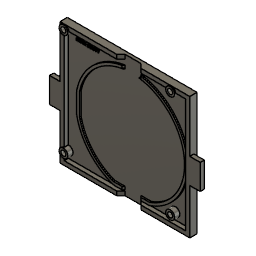
pin_grid_wafer_jig_sla (Autodesk Fusion 360 design; units mm, degrees)
part number: 2026-08-12-03-32-45-867
Autodesk Fusion 360 part; units mm, degrees
ref_plane "WorkPlane1" through (0, 0, 3) normal (0, 0, 1) x (1, 0, 0)
ref_plane "WorkPlane2" through (0, 0, 4.7) normal (0, 0, 1) x (1, 0, 0)
ref_plane "WorkPlane3" through (0, 0, 7.2) normal (0, 0, 1) x (1, 0, 0)
ref_plane "WorkPlane4" through (0, 0, 8) normal (0, 0, 1) x (1, 0, 0)
sketch "Wafer Platform Sketch" plane through (0, 0, 0) normal (0, 0, 1) x (1, 0, 0)
  line L0 (-55.05, -61.5817) -> (68.477, -61.5817)
  line L1 (68.477, -61.5817) -> (68.477, 55.05)
  line L2 (68.477, 55.05) -> (-55.05, 55.05)
  line L3 (-55.05, 55.05) -> (-55.05, -61.5817)
extrude "Wafer Platform" add sketch "Wafer Platform Sketch" along normal blind 3
sketch "4 x 4 mm Perimeter Reinforcement Bar Sketch" plane through (0, 0, 3) normal (0, 0, 1) x (1, 0, 0)
  line L0 (-55.05, -61.5817) -> (68.477, -61.5817)
  line L1 (68.477, -61.5817) -> (68.477, 55.05)
  line L2 (68.477, 55.05) -> (-55.05, 55.05)
  line L3 (-55.05, 55.05) -> (-55.05, -61.5817)
  line L4 (-51.05, -57.5817) -> (64.477, -57.5817)
  line L5 (64.477, -57.5817) -> (64.477, 51.05)
  line L6 (64.477, 51.05) -> (-51.05, 51.05)
  line L7 (-51.05, 51.05) -> (-51.05, -57.5817)
extrude "4 x 4 mm Perimeter Reinforcement Bar" add sketch "4 x 4 mm Perimeter Reinforcement Bar Sketch" along normal blind 4
sketch "Left Pickup Tab Sketch" plane through (0, 0, 3) normal (0, 0, 1) x (1, 0, 0)
  line L0 (-65.05, -18.296) -> (-55.05, -18.296)
  line L1 (-55.05, -18.296) -> (-55.05, 5.704)
  line L2 (-55.05, 5.704) -> (-65.05, 5.704)
  line L3 (-65.05, 5.704) -> (-65.05, -18.296)
extrude "Left Pickup Tab" add sketch "Left Pickup Tab Sketch" along normal blind 4
sketch "Right Pickup Tab Sketch" plane through (0, 0, 3) normal (0, 0, 1) x (1, 0, 0)
  line L0 (68.477, -18.296) -> (78.477, -18.296)
  line L1 (78.477, -18.296) -> (78.477, 5.704)
  line L2 (78.477, 5.704) -> (68.477, 5.704)
  line L3 (68.477, 5.704) -> (68.477, -18.296)
extrude "Right Pickup Tab" add sketch "Right Pickup Tab Sketch" along normal blind 4
sketch "15 mm Outer Bar Tweezer Notch with 45 Degree Sides Lower Sketch" plane through (0, 0, 3) normal (0, 0, 1) x (1, 0, 0)
  line L0 (2.977, -61.6817) -> (17.977, -61.6817)
  line L1 (17.977, -61.6817) -> (17.977, -57.4817)
  line L2 (17.977, -57.4817) -> (2.977, -57.4817)
  line L3 (2.977, -57.4817) -> (2.977, -61.6817)
sketch "15 mm Outer Bar Tweezer Notch with 45 Degree Sides Upper Sketch" plane through (0, 0, 7.2) normal (0, 0, 1) x (1, 0, 0)
  line L0 (-1.223, -65.8817) -> (22.177, -65.8817)
  line L1 (22.177, -65.8817) -> (22.177, -53.2817)
  line L2 (22.177, -53.2817) -> (-1.223, -53.2817)
  line L3 (-1.223, -53.2817) -> (-1.223, -65.8817)
loft "15 mm Outer Bar Tweezer Notch with 45 Degree Sides" cut profiles "15 mm Outer Bar Tweezer Notch with 45 Degree Sides Lower Sketch", "15 mm Outer Bar Tweezer Notch with 45 Degree Sides Upper Sketch" section 1 section 2
sketch "1.5 mm Raised Wafer Nest Sketch" plane through (0, 0, 3) normal (0, 0, 1) x (1, 0, 0)
  line L0 (63.477, -6.296) -> (63.4447, -4.4463)
  line L1 (63.4447, -4.4463) -> (63.3479, -2.5989)
  line L2 (63.3479, -2.5989) -> (63.1867, -0.756)
  line L3 (63.1867, -0.756) -> (62.9612, 1.0802)
  line L4 (62.9612, 1.0802) -> (62.6718, 2.9074)
  line L5 (62.6718, 2.9074) -> (62.3188, 4.7233)
  line L6 (62.3188, 4.7233) -> (61.9027, 6.5259)
  line L7 (61.9027, 6.5259) -> (61.4239, 8.3128)
  line L8 (61.4239, 8.3128) -> (60.883, 10.0819)
  line L9 (60.883, 10.0819) -> (60.2807, 11.8311)
  line L10 (60.2807, 11.8311) -> (59.6177, 13.5581)
  line L11 (59.6177, 13.5581) -> (58.8949, 15.261)
  line L12 (58.8949, 15.261) -> (58.1131, 16.9377)
  line L13 (58.1131, 16.9377) -> (57.2732, 18.586)
  line L14 (57.2732, 18.586) -> (56.3763, 20.204)
  line L15 (56.3763, 20.204) -> (55.4235, 21.7897)
  line L16 (55.4235, 21.7897) -> (54.416, 23.3412)
  line L17 (54.416, 23.3412) -> (53.3549, 24.8566)
  line L18 (53.3549, 24.8566) -> (52.2416, 26.3341)
  line L19 (52.2416, 26.3341) -> (51.0774, 27.7717)
  line L20 (51.0774, 27.7717) -> (49.8637, 29.1679)
  line L21 (49.8637, 29.1679) -> (48.602, 30.5209)
  line L22 (48.602, 30.5209) -> (47.2939, 31.829)
  line L23 (47.2939, 31.829) -> (45.9409, 33.0907)
  line L24 (45.9409, 33.0907) -> (44.5447, 34.3044)
  line L25 (44.5447, 34.3044) -> (43.1071, 35.4686)
  line L26 (43.1071, 35.4686) -> (41.6296, 36.5819)
  line L27 (41.6296, 36.5819) -> (40.1142, 37.643)
  line L28 (40.1142, 37.643) -> (38.5627, 38.6505)
  line L29 (38.5627, 38.6505) -> (36.977, 39.6033)
  line L30 (36.977, 39.6033) -> (35.359, 40.5002)
  line L31 (35.359, 40.5002) -> (33.7107, 41.3401)
  line L32 (33.7107, 41.3401) -> (32.034, 42.1219)
  line L33 (32.034, 42.1219) -> (30.3311, 42.8447)
  line L34 (30.3311, 42.8447) -> (28.6041, 43.5077)
  line L35 (28.6041, 43.5077) -> (26.8549, 44.11)
  line L36 (26.8549, 44.11) -> (25.0858, 44.6509)
  line L37 (25.0858, 44.6509) -> (23.2989, 45.1297)
  line L38 (23.2989, 45.1297) -> (21.4963, 45.5458)
  line L39 (21.4963, 45.5458) -> (19.6804, 45.8988)
  line L40 (19.6804, 45.8988) -> (17.8532, 46.1882)
  line L41 (17.8532, 46.1882) -> (16.017, 46.4137)
  line L42 (16.017, 46.4137) -> (14.1741, 46.5749)
  line L43 (14.1741, 46.5749) -> (12.3267, 46.6717)
  line L44 (12.3267, 46.6717) -> (10.477, 46.704)
  line L45 (10.477, 46.704) -> (8.6273, 46.6717)
  line L46 (8.6273, 46.6717) -> (6.7799, 46.5749)
  line L47 (6.7799, 46.5749) -> (4.937, 46.4137)
  line L48 (4.937, 46.4137) -> (3.1008, 46.1882)
  line L49 (3.1008, 46.1882) -> (1.2736, 45.8988)
  line L50 (1.2736, 45.8988) -> (-0.5423, 45.5458)
  line L51 (-0.5423, 45.5458) -> (-2.3449, 45.1297)
  line L52 (-2.3449, 45.1297) -> (-4.1318, 44.6509)
  line L53 (-4.1318, 44.6509) -> (-5.9009, 44.11)
  line L54 (-5.9009, 44.11) -> (-7.6501, 43.5077)
  line L55 (-7.6501, 43.5077) -> (-9.3771, 42.8447)
  line L56 (-9.3771, 42.8447) -> (-11.08, 42.1219)
  line L57 (-11.08, 42.1219) -> (-12.7567, 41.3401)
  line L58 (-12.7567, 41.3401) -> (-14.405, 40.5002)
  line L59 (-14.405, 40.5002) -> (-16.023, 39.6033)
  line L60 (-16.023, 39.6033) -> (-17.6087, 38.6505)
  line L61 (-17.6087, 38.6505) -> (-19.1602, 37.643)
  line L62 (-19.1602, 37.643) -> (-20.6756, 36.5819)
  line L63 (-20.6756, 36.5819) -> (-22.1531, 35.4686)
  line L64 (-22.1531, 35.4686) -> (-23.5907, 34.3044)
  line L65 (-23.5907, 34.3044) -> (-24.9869, 33.0907)
  line L66 (-24.9869, 33.0907) -> (-26.3399, 31.829)
  line L67 (-26.3399, 31.829) -> (-27.648, 30.5209)
  line L68 (-27.648, 30.5209) -> (-28.9097, 29.1679)
  line L69 (-28.9097, 29.1679) -> (-30.1234, 27.7717)
  line L70 (-30.1234, 27.7717) -> (-31.2876, 26.3341)
  line L71 (-31.2876, 26.3341) -> (-32.4009, 24.8566)
  line L72 (-32.4009, 24.8566) -> (-33.462, 23.3412)
  line L73 (-33.462, 23.3412) -> (-34.4695, 21.7897)
  line L74 (-34.4695, 21.7897) -> (-35.4223, 20.204)
  line L75 (-35.4223, 20.204) -> (-36.3192, 18.586)
  line L76 (-36.3192, 18.586) -> (-37.1591, 16.9377)
  line L77 (-37.1591, 16.9377) -> (-37.9409, 15.261)
  line L78 (-37.9409, 15.261) -> (-38.6637, 13.5581)
  line L79 (-38.6637, 13.5581) -> (-39.3267, 11.8311)
  line L80 (-39.3267, 11.8311) -> (-39.929, 10.0819)
  line L81 (-39.929, 10.0819) -> (-40.4699, 8.3128)
  line L82 (-40.4699, 8.3128) -> (-40.9487, 6.5259)
  line L83 (-40.9487, 6.5259) -> (-41.3648, 4.7233)
  line L84 (-41.3648, 4.7233) -> (-41.7063, 2.9664)
  line L85 (-41.7063, 2.9664) -> (-41.7063, -15.5584)
  line L86 (-41.7063, -15.5584) -> (-41.3648, -17.3153)
  line L87 (-41.3648, -17.3153) -> (-40.9487, -19.1179)
  line L88 (-40.9487, -19.1179) -> (-40.4699, -20.9048)
  line L89 (-40.4699, -20.9048) -> (-39.929, -22.6739)
  line L90 (-39.929, -22.6739) -> (-39.3267, -24.4231)
  line L91 (-39.3267, -24.4231) -> (-38.6637, -26.1501)
  line L92 (-38.6637, -26.1501) -> (-37.9409, -27.853)
  line L93 (-37.9409, -27.853) -> (-37.1591, -29.5297)
  line L94 (-37.1591, -29.5297) -> (-36.3192, -31.178)
  line L95 (-36.3192, -31.178) -> (-35.4223, -32.796)
  line L96 (-35.4223, -32.796) -> (-34.4695, -34.3817)
  line L97 (-34.4695, -34.3817) -> (-33.462, -35.9332)
  line L98 (-33.462, -35.9332) -> (-32.4009, -37.4486)
  line L99 (-32.4009, -37.4486) -> (-31.2876, -38.9261)
  line L100 (-31.2876, -38.9261) -> (-30.1234, -40.3637)
  line L101 (-30.1234, -40.3637) -> (-28.9097, -41.7599)
  line L102 (-28.9097, -41.7599) -> (-27.648, -43.1129)
  line L103 (-27.648, -43.1129) -> (-26.3399, -44.421)
  line L104 (-26.3399, -44.421) -> (-24.9869, -45.6827)
  line L105 (-24.9869, -45.6827) -> (-23.5907, -46.8964)
  line L106 (-23.5907, -46.8964) -> (-22.1531, -48.0606)
  line L107 (-22.1531, -48.0606) -> (-20.6756, -49.1739)
  line L108 (-20.6756, -49.1739) -> (-19.1602, -50.235)
  line L109 (-19.1602, -50.235) -> (-17.6087, -51.2425)
  line L110 (-17.6087, -51.2425) -> (-16.023, -52.1953)
  line L111 (-16.023, -52.1953) -> (-14.405, -53.0922)
  line L112 (-14.405, -53.0922) -> (-12.7567, -53.9321)
  line L113 (-12.7567, -53.9321) -> (-11.08, -54.7139)
  line L114 (-11.08, -54.7139) -> (-9.3771, -55.4367)
  line L115 (-9.3771, -55.4367) -> (-7.6501, -56.0997)
  line L116 (-7.6501, -56.0997) -> (-6.2503, -56.5817)
  line L117 (-6.2503, -56.5817) -> (27.2043, -56.5817)
  line L118 (27.2043, -56.5817) -> (28.6041, -56.0997)
  line L119 (28.6041, -56.0997) -> (30.3311, -55.4367)
  line L120 (30.3311, -55.4367) -> (32.034, -54.7139)
  line L121 (32.034, -54.7139) -> (33.7107, -53.9321)
  line L122 (33.7107, -53.9321) -> (35.359, -53.0922)
  line L123 (35.359, -53.0922) -> (36.977, -52.1953)
  line L124 (36.977, -52.1953) -> (38.5627, -51.2425)
  line L125 (38.5627, -51.2425) -> (40.1142, -50.235)
  line L126 (40.1142, -50.235) -> (41.6296, -49.1739)
  line L127 (41.6296, -49.1739) -> (43.1071, -48.0606)
  line L128 (43.1071, -48.0606) -> (44.5447, -46.8964)
  line L129 (44.5447, -46.8964) -> (45.9409, -45.6827)
  line L130 (45.9409, -45.6827) -> (47.2939, -44.421)
  line L131 (47.2939, -44.421) -> (48.602, -43.1129)
  line L132 (48.602, -43.1129) -> (49.8637, -41.7599)
  line L133 (49.8637, -41.7599) -> (51.0774, -40.3637)
  line L134 (51.0774, -40.3637) -> (52.2416, -38.9261)
  line L135 (52.2416, -38.9261) -> (53.3549, -37.4486)
  line L136 (53.3549, -37.4486) -> (54.416, -35.9332)
  line L137 (54.416, -35.9332) -> (55.4235, -34.3817)
  line L138 (55.4235, -34.3817) -> (56.3763, -32.796)
  line L139 (56.3763, -32.796) -> (57.2732, -31.178)
  line L140 (57.2732, -31.178) -> (58.1131, -29.5297)
  line L141 (58.1131, -29.5297) -> (58.8949, -27.853)
  line L142 (58.8949, -27.853) -> (59.6177, -26.1501)
  line L143 (59.6177, -26.1501) -> (60.2807, -24.4231)
  line L144 (60.2807, -24.4231) -> (60.883, -22.6739)
  line L145 (60.883, -22.6739) -> (61.4239, -20.9048)
  line L146 (61.4239, -20.9048) -> (61.9027, -19.1179)
  line L147 (61.9027, -19.1179) -> (62.3188, -17.3153)
  line L148 (62.3188, -17.3153) -> (62.6718, -15.4994)
  line L149 (62.6718, -15.4994) -> (62.9612, -13.6722)
  line L150 (62.9612, -13.6722) -> (63.1867, -11.836)
  line L151 (63.1867, -11.836) -> (63.3479, -9.9931)
  line L152 (63.3479, -9.9931) -> (63.4447, -8.1457)
  line L153 (63.4447, -8.1457) -> (63.477, -6.296)
extrude "1.5 mm Raised Wafer Nest" add sketch "1.5 mm Raised Wafer Nest Sketch" along normal blind 1.5
sketch "Final Wafer Pocket Clearance Sketch" plane through (0, 0, 3) normal (0, 0, 1) x (1, 0, 0)
  line L0 (60.977, -6.296) -> (60.9462, -4.5336)
  line L1 (60.9462, -4.5336) -> (60.854, -2.7733)
  line L2 (60.854, -2.7733) -> (60.7004, -1.0173)
  line L3 (60.7004, -1.0173) -> (60.4855, 0.7322)
  line L4 (60.4855, 0.7322) -> (60.2098, 2.4732)
  line L5 (60.2098, 2.4732) -> (59.8735, 4.2035)
  line L6 (59.8735, 4.2035) -> (59.4769, 5.9211)
  line L7 (59.4769, 5.9211) -> (59.0207, 7.6237)
  line L8 (59.0207, 7.6237) -> (58.5054, 9.3094)
  line L9 (58.5054, 9.3094) -> (57.9315, 10.976)
  line L10 (57.9315, 10.976) -> (57.2998, 12.6216)
  line L11 (57.2998, 12.6216) -> (56.611, 14.2442)
  line L12 (56.611, 14.2442) -> (55.8661, 15.8417)
  line L13 (55.8661, 15.8417) -> (55.0659, 17.4123)
  line L14 (55.0659, 17.4123) -> (54.2113, 18.954)
  line L15 (54.2113, 18.954) -> (53.3034, 20.4649)
  line L16 (53.3034, 20.4649) -> (52.3434, 21.9432)
  line L17 (52.3434, 21.9432) -> (51.3324, 23.3872)
  line L18 (51.3324, 23.3872) -> (50.2715, 24.7949)
  line L19 (50.2715, 24.7949) -> (49.1622, 26.1648)
  line L20 (49.1622, 26.1648) -> (48.0058, 27.4951)
  line L21 (48.0058, 27.4951) -> (46.8037, 28.7842)
  line L22 (46.8037, 28.7842) -> (45.5572, 30.0307)
  line L23 (45.5572, 30.0307) -> (44.2681, 31.2328)
  line L24 (44.2681, 31.2328) -> (42.9378, 32.3892)
  line L25 (42.9378, 32.3892) -> (41.5679, 33.4985)
  line L26 (41.5679, 33.4985) -> (40.1602, 34.5594)
  line L27 (40.1602, 34.5594) -> (38.7162, 35.5704)
  line L28 (38.7162, 35.5704) -> (37.2379, 36.5304)
  line L29 (37.2379, 36.5304) -> (35.727, 37.4383)
  line L30 (35.727, 37.4383) -> (34.1853, 38.2929)
  line L31 (34.1853, 38.2929) -> (32.6147, 39.0931)
  line L32 (32.6147, 39.0931) -> (31.0172, 39.838)
  line L33 (31.0172, 39.838) -> (29.3946, 40.5268)
  line L34 (29.3946, 40.5268) -> (27.749, 41.1585)
  line L35 (27.749, 41.1585) -> (26.0824, 41.7324)
  line L36 (26.0824, 41.7324) -> (24.3967, 42.2477)
  line L37 (24.3967, 42.2477) -> (22.6941, 42.7039)
  line L38 (22.6941, 42.7039) -> (20.9765, 43.1005)
  line L39 (20.9765, 43.1005) -> (19.2462, 43.4368)
  line L40 (19.2462, 43.4368) -> (17.5052, 43.7125)
  line L41 (17.5052, 43.7125) -> (15.7557, 43.9274)
  line L42 (15.7557, 43.9274) -> (13.9997, 44.081)
  line L43 (13.9997, 44.081) -> (12.2394, 44.1732)
  line L44 (12.2394, 44.1732) -> (10.477, 44.204)
  line L45 (10.477, 44.204) -> (8.7146, 44.1732)
  line L46 (8.7146, 44.1732) -> (6.9543, 44.081)
  line L47 (6.9543, 44.081) -> (5.1983, 43.9274)
  line L48 (5.1983, 43.9274) -> (3.4488, 43.7125)
  line L49 (3.4488, 43.7125) -> (1.7078, 43.4368)
  line L50 (1.7078, 43.4368) -> (-0.0225, 43.1005)
  line L51 (-0.0225, 43.1005) -> (-1.7401, 42.7039)
  line L52 (-1.7401, 42.7039) -> (-3.4427, 42.2477)
  line L53 (-3.4427, 42.2477) -> (-5.1284, 41.7324)
  line L54 (-5.1284, 41.7324) -> (-6.795, 41.1585)
  line L55 (-6.795, 41.1585) -> (-8.4406, 40.5268)
  line L56 (-8.4406, 40.5268) -> (-10.0632, 39.838)
  line L57 (-10.0632, 39.838) -> (-11.6607, 39.0931)
  line L58 (-11.6607, 39.0931) -> (-13.2313, 38.2929)
  line L59 (-13.2313, 38.2929) -> (-14.773, 37.4383)
  line L60 (-14.773, 37.4383) -> (-16.2839, 36.5304)
  line L61 (-16.2839, 36.5304) -> (-17.7622, 35.5704)
  line L62 (-17.7622, 35.5704) -> (-19.2062, 34.5594)
  line L63 (-19.2062, 34.5594) -> (-20.6139, 33.4985)
  line L64 (-20.6139, 33.4985) -> (-21.9838, 32.3892)
  line L65 (-21.9838, 32.3892) -> (-23.3141, 31.2328)
  line L66 (-23.3141, 31.2328) -> (-24.6032, 30.0307)
  line L67 (-24.6032, 30.0307) -> (-25.8497, 28.7842)
  line L68 (-25.8497, 28.7842) -> (-27.0518, 27.4951)
  line L69 (-27.0518, 27.4951) -> (-28.2082, 26.1648)
  line L70 (-28.2082, 26.1648) -> (-29.3175, 24.7949)
  line L71 (-29.3175, 24.7949) -> (-30.3784, 23.3872)
  line L72 (-30.3784, 23.3872) -> (-31.3894, 21.9432)
  line L73 (-31.3894, 21.9432) -> (-32.3494, 20.4649)
  line L74 (-32.3494, 20.4649) -> (-33.2573, 18.954)
  line L75 (-33.2573, 18.954) -> (-34.1119, 17.4123)
  line L76 (-34.1119, 17.4123) -> (-34.9121, 15.8417)
  line L77 (-34.9121, 15.8417) -> (-35.657, 14.2442)
  line L78 (-35.657, 14.2442) -> (-36.3458, 12.6216)
  line L79 (-36.3458, 12.6216) -> (-36.9775, 10.976)
  line L80 (-36.9775, 10.976) -> (-37.5514, 9.3094)
  line L81 (-37.5514, 9.3094) -> (-38.0667, 7.6237)
  line L82 (-38.0667, 7.6237) -> (-38.5229, 5.9211)
  line L83 (-38.5229, 5.9211) -> (-38.8813, 4.3687)
  line L84 (-38.8813, 4.3687) -> (-38.8813, -16.9607)
  line L85 (-38.8813, -16.9607) -> (-38.5229, -18.5131)
  line L86 (-38.5229, -18.5131) -> (-38.0667, -20.2157)
  line L87 (-38.0667, -20.2157) -> (-37.5514, -21.9014)
  line L88 (-37.5514, -21.9014) -> (-36.9775, -23.568)
  line L89 (-36.9775, -23.568) -> (-36.3458, -25.2136)
  line L90 (-36.3458, -25.2136) -> (-35.657, -26.8362)
  line L91 (-35.657, -26.8362) -> (-34.9121, -28.4337)
  line L92 (-34.9121, -28.4337) -> (-34.1119, -30.0043)
  line L93 (-34.1119, -30.0043) -> (-33.2573, -31.546)
  line L94 (-33.2573, -31.546) -> (-32.3494, -33.0569)
  line L95 (-32.3494, -33.0569) -> (-31.3894, -34.5352)
  line L96 (-31.3894, -34.5352) -> (-30.3784, -35.9792)
  line L97 (-30.3784, -35.9792) -> (-29.3175, -37.3869)
  line L98 (-29.3175, -37.3869) -> (-28.2082, -38.7568)
  line L99 (-28.2082, -38.7568) -> (-27.0518, -40.0871)
  line L100 (-27.0518, -40.0871) -> (-25.8497, -41.3762)
  line L101 (-25.8497, -41.3762) -> (-24.6032, -42.6227)
  line L102 (-24.6032, -42.6227) -> (-23.3141, -43.8248)
  line L103 (-23.3141, -43.8248) -> (-21.9838, -44.9812)
  line L104 (-21.9838, -44.9812) -> (-20.6139, -46.0905)
  line L105 (-20.6139, -46.0905) -> (-19.2062, -47.1514)
  line L106 (-19.2062, -47.1514) -> (-17.7622, -48.1624)
  line L107 (-17.7622, -48.1624) -> (-16.2839, -49.1224)
  line L108 (-16.2839, -49.1224) -> (-14.773, -50.0303)
  line L109 (-14.773, -50.0303) -> (-13.2313, -50.8849)
  line L110 (-13.2313, -50.8849) -> (-11.6607, -51.6851)
  line L111 (-11.6607, -51.6851) -> (-10.0632, -52.43)
  line L112 (-10.0632, -52.43) -> (-8.4406, -53.1188)
  line L113 (-8.4406, -53.1188) -> (-6.795, -53.7505)
  line L114 (-6.795, -53.7505) -> (-6.7769, -53.7567)
  line L115 (-6.7769, -53.7567) -> (27.7309, -53.7567)
  line L116 (27.7309, -53.7567) -> (27.749, -53.7505)
  line L117 (27.749, -53.7505) -> (29.3946, -53.1188)
  line L118 (29.3946, -53.1188) -> (31.0172, -52.43)
  line L119 (31.0172, -52.43) -> (32.6147, -51.6851)
  line L120 (32.6147, -51.6851) -> (34.1853, -50.8849)
  line L121 (34.1853, -50.8849) -> (35.727, -50.0303)
  line L122 (35.727, -50.0303) -> (37.2379, -49.1224)
  line L123 (37.2379, -49.1224) -> (38.7162, -48.1624)
  line L124 (38.7162, -48.1624) -> (40.1602, -47.1514)
  line L125 (40.1602, -47.1514) -> (41.5679, -46.0905)
  line L126 (41.5679, -46.0905) -> (42.9378, -44.9812)
  line L127 (42.9378, -44.9812) -> (44.2681, -43.8248)
  line L128 (44.2681, -43.8248) -> (45.5572, -42.6227)
  line L129 (45.5572, -42.6227) -> (46.8037, -41.3762)
  line L130 (46.8037, -41.3762) -> (48.0058, -40.0871)
  line L131 (48.0058, -40.0871) -> (49.1622, -38.7568)
  line L132 (49.1622, -38.7568) -> (50.2715, -37.3869)
  line L133 (50.2715, -37.3869) -> (51.3324, -35.9792)
  line L134 (51.3324, -35.9792) -> (52.3434, -34.5352)
  line L135 (52.3434, -34.5352) -> (53.3034, -33.0569)
  line L136 (53.3034, -33.0569) -> (54.2113, -31.546)
  line L137 (54.2113, -31.546) -> (55.0659, -30.0043)
  line L138 (55.0659, -30.0043) -> (55.8661, -28.4337)
  line L139 (55.8661, -28.4337) -> (56.611, -26.8362)
  line L140 (56.611, -26.8362) -> (57.2998, -25.2136)
  line L141 (57.2998, -25.2136) -> (57.9315, -23.568)
  line L142 (57.9315, -23.568) -> (58.5054, -21.9014)
  line L143 (58.5054, -21.9014) -> (59.0207, -20.2157)
  line L144 (59.0207, -20.2157) -> (59.4769, -18.5131)
  line L145 (59.4769, -18.5131) -> (59.8735, -16.7955)
  line L146 (59.8735, -16.7955) -> (60.2098, -15.0652)
  line L147 (60.2098, -15.0652) -> (60.4855, -13.3242)
  line L148 (60.4855, -13.3242) -> (60.7004, -11.5747)
  line L149 (60.7004, -11.5747) -> (60.854, -9.8187)
  line L150 (60.854, -9.8187) -> (60.9462, -8.0584)
  line L151 (60.9462, -8.0584) -> (60.977, -6.296)
extrude "Final Wafer Pocket Clearance" cut sketch "Final Wafer Pocket Clearance Sketch" along normal blind 1.6
sketch "15 mm Pickup Opening with 45 Degree Bevel Lower Sketch" plane through (0, 0, 3) normal (0, 0, 1) x (1, 0, 0)
  line L0 (2.977, -56.5817) -> (2.977, -53.5817)
  line L1 (2.977, -53.5817) -> (3.0242, -52.742)
  line L2 (3.0242, -52.742) -> (3.165, -51.9128)
  line L3 (3.165, -51.9128) -> (3.3979, -51.1046)
  line L4 (3.3979, -51.1046) -> (3.7197, -50.3276)
  line L5 (3.7197, -50.3276) -> (4.1266, -49.5915)
  line L6 (4.1266, -49.5915) -> (4.6133, -48.9055)
  line L7 (4.6133, -48.9055) -> (5.1737, -48.2784)
  line L8 (5.1737, -48.2784) -> (5.8008, -47.718)
  line L9 (5.8008, -47.718) -> (6.4868, -47.2313)
  line L10 (6.4868, -47.2313) -> (7.2229, -46.8244)
  line L11 (7.2229, -46.8244) -> (7.9999, -46.5026)
  line L12 (7.9999, -46.5026) -> (8.8081, -46.2697)
  line L13 (8.8081, -46.2697) -> (9.6373, -46.1289)
  line L14 (9.6373, -46.1289) -> (10.477, -46.0817)
  line L15 (10.477, -46.0817) -> (11.3167, -46.1289)
  line L16 (11.3167, -46.1289) -> (12.1459, -46.2697)
  line L17 (12.1459, -46.2697) -> (12.9541, -46.5026)
  line L18 (12.9541, -46.5026) -> (13.7311, -46.8244)
  line L19 (13.7311, -46.8244) -> (14.4672, -47.2313)
  line L20 (14.4672, -47.2313) -> (15.1532, -47.718)
  line L21 (15.1532, -47.718) -> (15.7803, -48.2784)
  line L22 (15.7803, -48.2784) -> (16.3407, -48.9055)
  line L23 (16.3407, -48.9055) -> (16.8274, -49.5915)
  line L24 (16.8274, -49.5915) -> (17.2343, -50.3276)
  line L25 (17.2343, -50.3276) -> (17.5561, -51.1046)
  line L26 (17.5561, -51.1046) -> (17.789, -51.9128)
  line L27 (17.789, -51.9128) -> (17.9298, -52.742)
  line L28 (17.9298, -52.742) -> (17.977, -53.5817)
  line L29 (17.977, -53.5817) -> (17.977, -56.5817)
  line L30 (17.977, -56.5817) -> (17.9298, -57.4214)
  line L31 (17.9298, -57.4214) -> (17.789, -58.2506)
  line L32 (17.789, -58.2506) -> (17.5561, -59.0588)
  line L33 (17.5561, -59.0588) -> (17.2343, -59.8358)
  line L34 (17.2343, -59.8358) -> (16.8274, -60.5719)
  line L35 (16.8274, -60.5719) -> (16.3407, -61.2579)
  line L36 (16.3407, -61.2579) -> (15.7803, -61.885)
  line L37 (15.7803, -61.885) -> (15.1532, -62.4454)
  line L38 (15.1532, -62.4454) -> (14.4672, -62.9321)
  line L39 (14.4672, -62.9321) -> (13.7311, -63.339)
  line L40 (13.7311, -63.339) -> (12.9541, -63.6608)
  line L41 (12.9541, -63.6608) -> (12.1459, -63.8937)
  line L42 (12.1459, -63.8937) -> (11.3167, -64.0345)
  line L43 (11.3167, -64.0345) -> (10.477, -64.0817)
  line L44 (10.477, -64.0817) -> (9.6373, -64.0345)
  line L45 (9.6373, -64.0345) -> (8.8081, -63.8937)
  line L46 (8.8081, -63.8937) -> (7.9999, -63.6608)
  line L47 (7.9999, -63.6608) -> (7.2229, -63.339)
  line L48 (7.2229, -63.339) -> (6.4868, -62.9321)
  line L49 (6.4868, -62.9321) -> (5.8008, -62.4454)
  line L50 (5.8008, -62.4454) -> (5.1737, -61.885)
  line L51 (5.1737, -61.885) -> (4.6133, -61.2579)
  line L52 (4.6133, -61.2579) -> (4.1266, -60.5719)
  line L53 (4.1266, -60.5719) -> (3.7197, -59.8358)
  line L54 (3.7197, -59.8358) -> (3.3979, -59.0588)
  line L55 (3.3979, -59.0588) -> (3.165, -58.2506)
  line L56 (3.165, -58.2506) -> (3.0242, -57.4214)
  line L57 (3.0242, -57.4214) -> (2.977, -56.5817)
sketch "15 mm Pickup Opening with 45 Degree Bevel Upper Sketch" plane through (0, 0, 4.7) normal (0, 0, 1) x (1, 0, 0)
  line L0 (1.277, -58.2817) -> (1.277, -51.8817)
  line L1 (1.277, -51.8817) -> (1.3348, -50.8516)
  line L2 (1.3348, -50.8516) -> (1.5077, -49.8345)
  line L3 (1.5077, -49.8345) -> (1.7933, -48.8431)
  line L4 (1.7933, -48.8431) -> (2.1881, -47.89)
  line L5 (2.1881, -47.89) -> (2.6871, -46.987)
  line L6 (2.6871, -46.987) -> (3.2842, -46.1456)
  line L7 (3.2842, -46.1456) -> (3.9716, -45.3763)
  line L8 (3.9716, -45.3763) -> (4.7409, -44.6889)
  line L9 (4.7409, -44.6889) -> (5.5823, -44.0918)
  line L10 (5.5823, -44.0918) -> (6.4853, -43.5928)
  line L11 (6.4853, -43.5928) -> (7.4384, -43.198)
  line L12 (7.4384, -43.198) -> (8.4298, -42.9124)
  line L13 (8.4298, -42.9124) -> (9.4469, -42.7395)
  line L14 (9.4469, -42.7395) -> (10.477, -42.6817)
  line L15 (10.477, -42.6817) -> (11.5071, -42.7395)
  line L16 (11.5071, -42.7395) -> (12.5242, -42.9124)
  line L17 (12.5242, -42.9124) -> (13.5156, -43.198)
  line L18 (13.5156, -43.198) -> (14.4687, -43.5928)
  line L19 (14.4687, -43.5928) -> (15.3717, -44.0918)
  line L20 (15.3717, -44.0918) -> (16.2131, -44.6889)
  line L21 (16.2131, -44.6889) -> (16.9824, -45.3763)
  line L22 (16.9824, -45.3763) -> (17.6698, -46.1456)
  line L23 (17.6698, -46.1456) -> (18.2669, -46.987)
  line L24 (18.2669, -46.987) -> (18.7659, -47.89)
  line L25 (18.7659, -47.89) -> (19.1607, -48.8431)
  line L26 (19.1607, -48.8431) -> (19.4463, -49.8345)
  line L27 (19.4463, -49.8345) -> (19.6192, -50.8516)
  line L28 (19.6192, -50.8516) -> (19.677, -51.8817)
  line L29 (19.677, -51.8817) -> (19.677, -58.2817)
  line L30 (19.677, -58.2817) -> (19.6192, -59.3118)
  line L31 (19.6192, -59.3118) -> (19.4463, -60.3289)
  line L32 (19.4463, -60.3289) -> (19.1607, -61.3203)
  line L33 (19.1607, -61.3203) -> (18.7659, -62.2734)
  line L34 (18.7659, -62.2734) -> (18.2669, -63.1764)
  line L35 (18.2669, -63.1764) -> (17.6698, -64.0178)
  line L36 (17.6698, -64.0178) -> (16.9824, -64.7871)
  line L37 (16.9824, -64.7871) -> (16.2131, -65.4746)
  line L38 (16.2131, -65.4746) -> (15.3717, -66.0716)
  line L39 (15.3717, -66.0716) -> (14.4687, -66.5706)
  line L40 (14.4687, -66.5706) -> (13.5156, -66.9654)
  line L41 (13.5156, -66.9654) -> (12.5242, -67.251)
  line L42 (12.5242, -67.251) -> (11.5071, -67.4239)
  line L43 (11.5071, -67.4239) -> (10.477, -67.4817)
  line L44 (10.477, -67.4817) -> (9.4469, -67.4239)
  line L45 (9.4469, -67.4239) -> (8.4298, -67.251)
  line L46 (8.4298, -67.251) -> (7.4384, -66.9654)
  line L47 (7.4384, -66.9654) -> (6.4853, -66.5706)
  line L48 (6.4853, -66.5706) -> (5.5823, -66.0716)
  line L49 (5.5823, -66.0716) -> (4.7409, -65.4746)
  line L50 (4.7409, -65.4746) -> (3.9716, -64.7871)
  line L51 (3.9716, -64.7871) -> (3.2842, -64.0178)
  line L52 (3.2842, -64.0178) -> (2.6871, -63.1764)
  line L53 (2.6871, -63.1764) -> (2.1881, -62.2734)
  line L54 (2.1881, -62.2734) -> (1.7933, -61.3203)
  line L55 (1.7933, -61.3203) -> (1.5077, -60.3289)
  line L56 (1.5077, -60.3289) -> (1.3348, -59.3118)
  line L57 (1.3348, -59.3118) -> (1.277, -58.2817)
loft "15 mm Pickup Opening with 45 Degree Bevel" cut profiles "15 mm Pickup Opening with 45 Degree Bevel Lower Sketch", "15 mm Pickup Opening with 45 Degree Bevel Upper Sketch" section 1 section 2
sketch "15 mm Rear Tape Gap with 45 Degree Bevel Lower Sketch" plane through (0, 0, 3) normal (0, 0, 1) x (1, 0, 0)
  line L0 (2.977, 43.704) -> (17.977, 43.704)
  line L1 (17.977, 43.704) -> (17.977, 46.904)
  line L2 (17.977, 46.904) -> (2.977, 46.904)
  line L3 (2.977, 46.904) -> (2.977, 43.704)
sketch "15 mm Rear Tape Gap with 45 Degree Bevel Upper Sketch" plane through (0, 0, 4.7) normal (0, 0, 1) x (1, 0, 0)
  line L0 (1.277, 43.704) -> (19.677, 43.704)
  line L1 (19.677, 43.704) -> (19.677, 46.904)
  line L2 (19.677, 46.904) -> (1.277, 46.904)
  line L3 (1.277, 46.904) -> (1.277, 43.704)
loft "15 mm Rear Tape Gap with 45 Degree Bevel" cut profiles "15 mm Rear Tape Gap with 45 Degree Bevel Lower Sketch", "15 mm Rear Tape Gap with 45 Degree Bevel Upper Sketch" section 1 section 2
sketch "15 mm Rear Outer Bar Notch with 45 Degree Sides Lower Sketch" plane through (0, 0, 3) normal (0, 0, 1) x (1, 0, 0)
  line L0 (2.977, 50.95) -> (17.977, 50.95)
  line L1 (17.977, 50.95) -> (17.977, 55.15)
  line L2 (17.977, 55.15) -> (2.977, 55.15)
  line L3 (2.977, 55.15) -> (2.977, 50.95)
sketch "15 mm Rear Outer Bar Notch with 45 Degree Sides Upper Sketch" plane through (0, 0, 7.2) normal (0, 0, 1) x (1, 0, 0)
  line L0 (-1.223, 46.75) -> (22.177, 46.75)
  line L1 (22.177, 46.75) -> (22.177, 59.35)
  line L2 (22.177, 59.35) -> (-1.223, 59.35)
  line L3 (-1.223, 59.35) -> (-1.223, 46.75)
loft "15 mm Rear Outer Bar Notch with 45 Degree Sides" cut profiles "15 mm Rear Outer Bar Notch with 45 Degree Sides Lower Sketch", "15 mm Rear Outer Bar Notch with 45 Degree Sides Upper Sketch" section 1 section 2
sketch "Outer Front Left Dowel Boss Sketch" plane through (0, 0, 3) normal (0, 0, 1) x (1, 0, 0)
  circle A0 centre (-50.8, -50.8) radius 4.25
extrude "Outer Front Left Dowel Boss" add sketch "Outer Front Left Dowel Boss Sketch" along normal blind 5
sketch "Outer Front Left Dowel Bore Sketch" plane through (0, 0, 8) normal (0, 0, 1) x (1, 0, 0)
  circle A0 centre (-50.8, -50.8) radius 2.4
extrude "Outer Front Left Dowel Bore" cut sketch "Outer Front Left Dowel Bore Sketch" against normal blind 8
sketch "Outer Front Right Dowel Boss Sketch" plane through (0, 0, 3) normal (0, 0, 1) x (1, 0, 0)
  circle A0 centre (50.8, -50.8) radius 4.25
extrude "Outer Front Right Dowel Boss" add sketch "Outer Front Right Dowel Boss Sketch" along normal blind 5
sketch "Outer Front Right Dowel Bore Sketch" plane through (0, 0, 8) normal (0, 0, 1) x (1, 0, 0)
  circle A0 centre (50.8, -50.8) radius 2.4
extrude "Outer Front Right Dowel Bore" cut sketch "Outer Front Right Dowel Bore Sketch" against normal blind 8
sketch "Outer Rear Left Dowel Boss Sketch" plane through (0, 0, 3) normal (0, 0, 1) x (1, 0, 0)
  circle A0 centre (-50.8, 50.8) radius 4.25
extrude "Outer Rear Left Dowel Boss" add sketch "Outer Rear Left Dowel Boss Sketch" along normal blind 5
sketch "Outer Rear Left Dowel Bore Sketch" plane through (0, 0, 8) normal (0, 0, 1) x (1, 0, 0)
  circle A0 centre (-50.8, 50.8) radius 2.4
extrude "Outer Rear Left Dowel Bore" cut sketch "Outer Rear Left Dowel Bore Sketch" against normal blind 8
sketch "Outer Rear Right Dowel Boss Sketch" plane through (0, 0, 3) normal (0, 0, 1) x (1, 0, 0)
  circle A0 centre (50.8, 50.8) radius 4.25
extrude "Outer Rear Right Dowel Boss" add sketch "Outer Rear Right Dowel Boss Sketch" along normal blind 5
sketch "Outer Rear Right Dowel Bore Sketch" plane through (0, 0, 8) normal (0, 0, 1) x (1, 0, 0)
  circle A0 centre (50.8, 50.8) radius 2.4
extrude "Outer Rear Right Dowel Bore" cut sketch "Outer Rear Right Dowel Bore Sketch" against normal blind 8
sketch "Designed By - 0.5 mm Engraving Sketch" plane through (0, 0, 3) normal (0, 0, 1) x (1, 0, 0)
  line L0 (-43.05, 36.05) -> (-3.05, 36.05) construction
  line L1 (-3.05, 36.05) -> (-3.05, 50.05) construction
  line L2 (-3.05, 50.05) -> (-43.05, 50.05) construction
  line L3 (-43.05, 50.05) -> (-43.05, 36.05) construction
  dimension "d56" = 2.5
  text T0 "DESIGNED BY:\nRYAN SCOTT" font "Arial" height 2.5 align left top in box 40 x 14 at (-43.05, 36.05) x (1, 0) y (0, 1) spacing 1 kerned
extrude "Designed By - 0.5 mm Engraving" add sketch "Designed By - 0.5 mm Engraving Sketch" along normal blind 0.5 text T0
equation "gridPitch = 25.4 mm" comment "Table hole-grid pitch"
equation "indexMove = 50.8 mm" comment "Two-grid-space indexing move"
equation "outerPinPatternSpan = 101.6 mm" comment "Four-space outer pin span"
equation "dowelDiameter = 4.7625 mm" comment "3/16 in steel locating dowel diameter"
equation "dowelHoleDiameter = 4.8 mm" comment "Press-fit bore for the dowel"
equation "bossHeight = 5.0 mm" comment "Dowel boss height above platform"
equation "bossDiameter = 8.5 mm" comment "Dowel boss outer diameter"
equation "platformSizeX = 123.527 mm" comment "Overall plate width"
equation "platformSizeY = 116.63170079844434 mm" comment "Overall plate depth"
equation "baseThickness = 3.0 mm" comment "Wafer platform thickness"
equation "outerBarWidth = 4.0 mm" comment "Perimeter reinforcement width"
equation "outerBarHeight = 4.0 mm" comment "Perimeter reinforcement height"
equation "sidewallHeight = 1.5 mm" comment "Nest lip height above platform"
equation "nestOffsetX = 7.29 mm" comment "Nest X from pin-square center"
equation "nestOffsetY = -4.95 mm" comment "Nest Y from pin-square center"
equation "pickupGapWidth = 15.0 mm" comment "Primary-flat pickup opening"
equation "rearTapeGapWidth = 15.0 mm" comment "Rear tape-access gap in the lip"
equation "annotationDepth = 0.5 mm" comment "Baseplate text engraving depth"
equation "annotationTextHeight = 2.5 mm" comment "Baseplate text height"
equation "d57 = 'DESIGNED BY:\\nRYAN SCOTT'"
